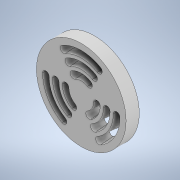
# Autodesk Inventor part: Мой ограничитель
Saved by Autodesk Inventor 2021 (Build 250183000, 183)
## iProperties
Created: 2020-11-07
Part Number: Мой ограничитель
Material: Типовые
Document SubType Name: Modeling
Designer: Тимоха
Density: 1 g/cm^3
Appearance: По умолчанию
Author: Тимоха
Autodesk Inventor part; units mm, degrees
ref_plane "YZ Plane" through (0, 0, 0) normal (1, 0, 0) x (0, 1, 0)
ref_plane "XZ Plane" through (0, 0, 0) normal (0, 1, 0) x (-1, 0, 0)
ref_plane "XY Plane" through (0, 0, 0) normal (0, 0, 1) x (1, 0, 0)
sketch "Эскиз1" plane through (0, 0, 0) normal (0, 0, 1) x (1, 0, 0)
  circle A0 centre (0, 0) radius 68
  dimension "d0" = 136
  constraints: 1 centre point, 1 coincident
  measures "d0" diameter of A0
extrude "Выдавливание1" add sketch "Эскиз1" along normal blind 20
sketch "Эскиз2" plane through (0, 0, 0) normal (0, 0, -1) x (-1, 0, 0)
  circle A0 centre (0, 0) radius 20
  dimension "d3" = 40
  constraints: 1 centre point, 1 coincident
  measures "d3" diameter of A0
extrude "Выдавливание2" add sketch "Эскиз2" along normal blind 6.5
sketch "Эскиз4" plane through (0, 0, 20) normal (0, 0, 1) x (1, 0, 0)
  circle A0 centre (0, 0) radius 20 projected
  circle A1 centre (0, 0) radius 68 projected
  circle A2 centre (0, 0) radius 20 projected
  arc A3 (9.375, 16.238) -> (14.375, 24.8982) centre (11.875, 20.5681) ccw
  arc A4 (17.0187, 29.1477) -> (22.0737, 37.7732) centre (19.6413, 33.4047) ccw
  arc A5 (24.375, 42.2187) -> (29.375, 50.879) centre (26.875, 46.5489) ccw
  arc A6 (9.375, 16.238) -> (-9.375, 16.238) centre (0, 0) ccw
  arc A7 (17.0187, 29.1477) -> (-17.1076, 29.0956) centre (0, 0) ccw
  arc A8 (24.375, 42.2187) -> (-24.375, 42.2187) centre (0, 0) ccw
  arc A9 (14.375, 24.8982) -> (-14.375, 24.8982) centre (0, 0) ccw
  arc A10 (22.276, 37.6542) -> (-22.175, 37.7138) centre (0, 0) ccw
  arc A11 (29.375, 50.879) -> (-29.375, 50.879) centre (0, 0) ccw
  arc A12 (-22.175, 37.7138) -> (-17.1076, 29.0956) centre (-19.6413, 33.4047) ccw
  arc A13 (-29.375, 50.879) -> (-24.375, 42.2187) centre (-26.875, 46.5489) ccw
  arc A14 (-14.375, 24.8982) -> (-9.375, 16.238) centre (-11.875, 20.5681) ccw
  arc A15 (-58.75, 0) -> (-29.375, -50.879) centre (0, 0) ccw
  arc A16 (-29.375, -50.879) -> (-24.375, -42.2187) centre (-26.875, -46.5489) ccw
  arc A17 (-48.75, 0) -> (-24.375, -42.2187) centre (0, 0) ccw
  arc A18 (-48.75, 0) -> (-58.75, 0) centre (-53.75, 0) ccw
  arc A19 (-33.752, 0.1647) -> (-43.7494, 0.2298) centre (-38.75, 0.3075) ccw
  arc A20 (-33.752, 0.1647) -> (-16.6437, -29.3635) centre (0, 0) ccw
  arc A21 (-21.5737, -38.061) -> (-16.6437, -29.3635) centre (-19.1087, -33.7122) ccw
  arc A22 (-43.7475, 0.4645) -> (-21.5737, -38.061) centre (0, 0) ccw
  arc A23 (-28.75, 0) -> (-14.375, -24.8982) centre (0, 0) ccw
  arc A24 (-14.375, -24.8982) -> (-9.375, -16.238) centre (-11.875, -20.5681) ccw
  arc A25 (-18.75, 0) -> (-9.375, -16.238) centre (0, 0) ccw
  arc A26 (-18.75, 0) -> (-28.75, 0) centre (-23.75, 0) ccw
  arc A27 (29.375, -50.879) -> (58.75, 0) centre (0, 0) ccw
  arc A28 (58.75, 0) -> (48.75, 0) centre (53.75, 0) ccw
  arc A29 (24.375, -42.2187) -> (48.75, 0) centre (0, 0) ccw
  arc A30 (24.375, -42.2187) -> (29.375, -50.879) centre (26.875, -46.5489) ccw
  arc A31 (16.7333, -29.3125) -> (21.6757, -38.003) centre (19.1087, -33.7122) ccw
  arc A32 (16.7333, -29.3125) -> (33.7514, 0.2678) centre (0, 0) ccw
  arc A33 (43.7486, 0.3472) -> (33.7514, 0.2678) centre (38.75, 0.3075) ccw
  arc A34 (21.4715, -38.1187) -> (43.7486, 0.3472) centre (0, 0) ccw
  arc A35 (14.375, -24.8982) -> (28.75, 0) centre (0, 0) ccw
  arc A36 (28.75, 0) -> (18.75, 0) centre (23.75, 0) ccw
  arc A37 (9.375, -16.238) -> (18.75, 0) centre (0, 0) ccw
  arc A38 (9.375, -16.238) -> (14.375, -24.8982) centre (11.875, -20.5681) ccw
  dimension "d18" = 10
  dimension "d19" = 10
  dimension "d20" = 10
  dimension "d21" = 57.5
  dimension "d22" = 87.5
  dimension "d26" = 360
  constraints: 78 point on circle, 36 centre point, 22 coincident, 7 tangent, 112 other
  measures "d18" diameter of A3
  measures "d19" diameter of A4
  measures "d20" diameter of A5
  measures "d21" diameter of A9
  measures "d22" diameter of A10
sketch "Эскиз3" plane through (0, 0, 0) normal (0, 0, -1) x (-1, 0, 0)
  arc A0 (10, 17.3205) -> (13.75, 23.8157) centre (11.875, 20.5681) ccw
  arc A1 (17.5, 30.3109) -> (21.25, 36.8061) centre (19.6413, 33.4047) ccw
  arc A2 (25, 43.3013) -> (28.75, 49.7965) centre (26.875, 46.5489) ccw
  arc A3 (-13.75, 23.8157) -> (-10, 17.3205) centre (-11.875, 20.5681) ccw
  arc A4 (-21.25, 36.8061) -> (-17.5, 30.3109) centre (-19.6413, 33.4047) ccw
  arc A5 (-28.75, 49.7965) -> (-25, 43.3013) centre (-26.875, 46.5489) ccw
  arc A6 (25, 43.3013) -> (-25, 43.3013) centre (0, 0) ccw
  arc A7 (28.75, 49.7965) -> (-28.75, 49.7965) centre (0, 0) ccw
  arc A8 (21.8314, 36.4642) -> (-21.8314, 36.4642) centre (0, 0) ccw
  arc A9 (17.9788, 30.0294) -> (-17.9788, 30.0294) centre (0, 0) ccw
  arc A10 (13.75, 23.8157) -> (-13.75, 23.8157) centre (0, 0) ccw
  arc A11 (10, -17.3205) -> (13.75, -23.8157) centre (11.875, -20.5681) ccw
  arc A12 (13.75, -23.8157) -> (27.5, 0) centre (0, 0) ccw
  arc A13 (27.5, 0) -> (20, 0) centre (23.75, 0) ccw
  arc A14 (42.5, 0) -> (35, 0) centre (38.75, 0.3075) ccw
  arc A15 (57.5, 0) -> (50, 0) centre (53.75, 0) ccw
  arc A16 (17.0168, -30.5848) -> (34.9956, 0.5554) centre (0, 0) ccw
  arc A17 (17.5, -30.3109) -> (21.25, -36.8061) centre (19.1087, -33.7122) ccw
  arc A18 (20.6632, -37.1387) -> (42.4946, 0.6744) centre (0, 0) ccw
  arc A19 (25, -43.3013) -> (50, 0) centre (0, 0) ccw
  arc A20 (25, -43.3013) -> (28.75, -49.7965) centre (26.875, -46.5489) ccw
  arc A21 (28.75, -49.7965) -> (57.5, 0) centre (0, 0) ccw
  arc A22 (-20, 0) -> (-27.5, 0) centre (-23.75, 0) ccw
  arc A23 (-27.5, 0) -> (-13.75, -23.8157) centre (0, 0) ccw
  arc A24 (-13.75, -23.8157) -> (-10, -17.3205) centre (-11.875, -20.5681) ccw
  arc A25 (-21.25, -36.8061) -> (-17.5, -30.3109) centre (-19.1087, -33.7122) ccw
  arc A26 (-28.75, -49.7965) -> (-25, -43.3013) centre (-26.875, -46.5489) ccw
  arc A27 (-34.9956, 0.5554) -> (-17.0168, -30.5848) centre (0, 0) ccw
  arc A28 (-35, 0) -> (-42.5, 0) centre (-38.75, 0.3075) ccw
  arc A29 (-42.4946, 0.6744) -> (-20.6632, -37.1387) centre (0, 0) ccw
  arc A30 (-50, 0) -> (-25, -43.3013) centre (0, 0) ccw
  arc A31 (-50, 0) -> (-57.5, 0) centre (-53.75, 0) ccw
  arc A32 (-57.5, 0) -> (-28.75, -49.7965) centre (0, 0) ccw
  arc A33 (10, -17.3205) -> (20, 0) centre (0, 0) ccw
  arc A34 (-20, 0) -> (-10, -17.3205) centre (0, 0) ccw
  arc A35 (10, 17.3205) -> (-10, 17.3205) centre (0, 0) ccw
  dimension "d12" = 3.75
  dimension "d13" = 3.7626
  dimension "d16" = 360
  constraints: 91 point on circle, 36 centre point, 20 coincident, 122 other
  measures "d12" radius of A0
  measures "d13" radius of A1
loft "Лофт1" cut profiles "Эскиз4", "Эскиз3" contours A0 A38 A37 A36 | A0 A36 A35 A38 / A34 A24 A23 A22
loft "Лофт2" cut profiles "Эскиз3", "Эскиз4" contours A29 A28 A27 A25 / A32 A33 A34 A31
loft "Лофт3" cut profiles "Эскиз4", "Эскиз3" contours A30 A29 A28 A27 / A32 A31 A30 A26
pattern_circular "Круговой массив1" count 3 over 360 about axis through (0, 0, -10) along (0, 0, 1) of "Лофт3", "Лофт2", "Лофт1"
